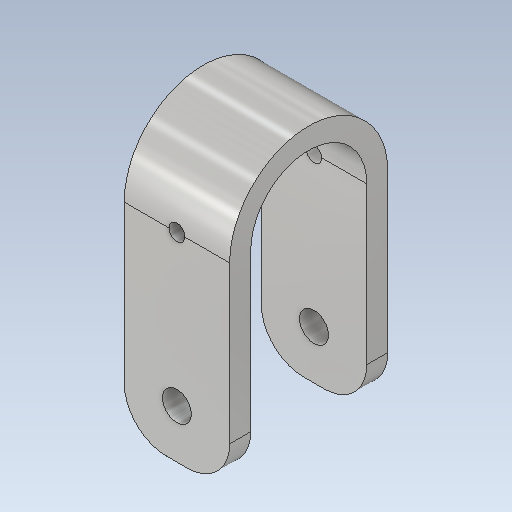
# Autodesk Inventor part: actuator_bracket1
Saved by Autodesk Inventor 2020 (Build 240168000, 168)
## iProperties
Created: 2017-11-30
Part Number: actuator_bracket1
Material: Generic
Document SubType Name: Modeling
Designer: stedrock
Density: 1 g/cm^3
Appearance: Default
Mass: 8.8362 g
Surface Area: 56.6716 cm^2
Volume: 8.8362 cm^3
Author: stedrock
Autodesk Inventor part; units mm, degrees
ref_plane "YZ Plane" through (0, 0, 0) normal (1, 0, 0) x (0, 1, 0)
ref_plane "XZ Plane" through (0, 0, 0) normal (0, 1, 0) x (-1, 0, 0)
ref_plane "XY Plane" through (0, 0, 0) normal (0, 0, 1) x (1, 0, 0)
sketch "Sketch1" plane through (0, 0, 0) normal (0, 1, 0) x (-1, 0, 0)
  line L0 (-10, 55) -> (10, 55)
  line L1 (10, 55) -> (10, -55)
  line L2 (10, -55) -> (-10, -55)
  line L3 (-10, -55) -> (-10, 55)
  line L4 (-10, 55) -> (10, -55) construction
  line L5 (10, 55) -> (-10, -55) construction
  line L6 (0, 0) -> (20.0722, 0)
  dimension "d0" = 20
  dimension "d1" = 110
  constraints: 14 end point, 2 horizontal, 2 midpoint, 2 parallel, 1 perpendicular
  measures "d0" distance of L1.end L2.end
  measures "d1" distance of L0.end L1.end
extrude "Extrusion1" add sketch "Sketch1" along normal blind 4
bend part "Bend Part1" radius 11 angle 180 line through (0, 0, 0) along (-1, 0, 0) centre toward (0, -1, 0) moving side (0, 0, 1) both sides yes
sketch "Sketch2" plane through (0, 0, 0) normal (0, 0, 1) x (1, 0, 0)
  line L0 (0, 0) -> (0, -71.9842) construction
  circle A0 centre (0, -39.5) radius 2.75
  circle A1 centre (0, -11) radius 1.5
  dimension "d6" = 5.5
  dimension "d7" = 39.5
  dimension "d11" = 3
  dimension "d12" = 11
  constraints: 2 centre point, 2 end point, 2 point on line, 1 vertical
  measures "d6" diameter of A0
  measures "d7" distance of A0.centre L0.start
  measures "d11" diameter of A1
  measures "d12" distance of L0.start A1.centre
extrude "holes" cut sketch "Sketch2" along normal through all both and the other way through all
fillet "Fillet1" radius 8 4 edges at (10, -48.7212, -13) (-10, -48.7212, -13) (-10, -48.7212, 13) (10, -48.7212, 13)
body "Solid1"
